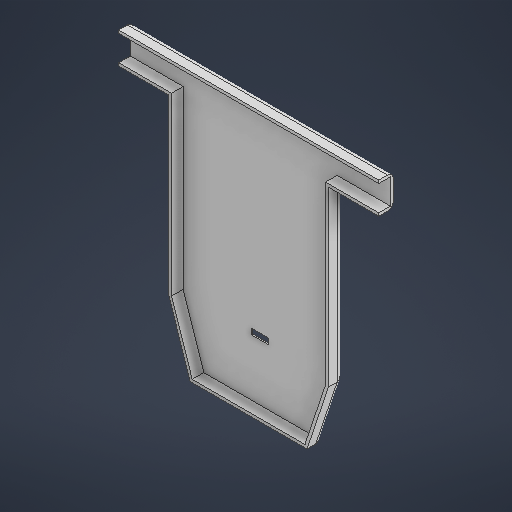
# Autodesk Inventor part: 8.7_수정본
Saved by Autodesk Inventor 2026 (Build 300175000, 175)
## iProperties
Created: 2025-08-07
Part Number: 8.7_수정본
Material: 일반
Document SubType Name: Modeling
Designer: rlarj
Density: 1 g/cm^3
Appearance: 기본값
Author: rlarj
Autodesk Inventor part; units mm, degrees
ref_plane "YZ Plane" through (0, 0, 0) normal (1, 0, 0) x (0, 1, 0)
ref_plane "XZ Plane" through (0, 0, 0) normal (0, 1, 0) x (-1, 0, 0)
ref_plane "XY Plane" through (0, 0, 0) normal (0, 0, 1) x (1, 0, 0)
sketch "스케치18" plane through (0, 0, 0) normal (0, 0, 1) x (1, 0, 0)
  line L0 (55, 0) -> (55, 20)
  line L1 (55, 20) -> (89.63, 20)
  line L2 (89.63, 20) -> (89.63, 41.5)
  line L3 (89.63, 41.5) -> (-89.4, 41.5)
  line L4 (-89.4, 41.5) -> (-89.4, 20)
  line L5 (-89.4, 20) -> (-55, 20)
  line L6 (-55, 20) -> (-55, -55)
  line L7 (55, 0) -> (55, -55)
  line L8 (-55, -55) -> (-55, -99.24)
  line L9 (-55, -99.24) -> (-40.255, -143.4879)
  line L10 (-40.255, -143.4879) -> (40.245, -143.4879)
  line L11 (55, -55) -> (55, -99.24)
  line L12 (55, -99.24) -> (40.245, -143.4879)
  point P0 (0, 0)
  dimension "d111" = 179.03
  dimension "d112" = 184.9879
  dimension "d113" = 34.4
  constraints: 26 end point, 5 vertical, 4 perpendicular, 2 point on line, 1 horizontal
  measures "d111" distance of L2.end L3.end
  measures "d112" vertical distance of L9.end L3.end
  measures "d113" distance of L4.end L5.end
extrude "돌출13" add sketch "스케치18" along normal blind 10
shell "쉘4" thickness 2 removed faces 1 at (-18.3333, -11.6667, 10)
sketch "스케치23" plane through (87.63, 22, 2) normal (-1, 0, 0) x (0, 0, 1)
  line L0 (0, 0) -> (8, 0) projected
  line L1 (0, 0) -> (0, 17.5) projected
  line L2 (8, 0) -> (0, 0)
  line L3 (0, 0) -> (0, 17.5)
  line L4 (0, 17.5) -> (8, 17.5)
  line L5 (8, 17.5) -> (8, 0)
  point P0 (-2, -22)
  constraints: 8 end point, 3 perpendicular, 1 collinear
extrude "돌출16" cut sketch "스케치23" along normal mid plane 600
fillet "모깎기6" radius 4 8 edges at (0.115, 41.5, 0) (72.315, 20, 0) (-72.2, 20, 0) (-55, -39.62, 0) (55, -39.62, 0) (47.6225, -121.3639, 0) (-0.005, -143.4879, 0) (-47.6275, -121.3639, 0)
sketch "스케치24" plane through (0, 0, 0) normal (0, 0, -1) x (-1, 0, 0)
  line L0 (0, -98.5907) -> (-13.5, -98.5907)
  line L1 (0, -98.5907) -> (13.5, -98.5907)
  line L2 (-13.5, -98.5907) -> (-13.5, -128.5907)
  line L3 (-13.5, -128.5907) -> (0, -128.5907)
  line L4 (0, -128.5907) -> (13.5, -128.5907)
  line L5 (13.5, -128.5907) -> (13.5, -98.5907)
  line L6 (0, -98.5907) -> (6, -98.5907)
  line L7 (6, -98.5907) -> (6, -102.5907)
  line L8 (6, -102.5907) -> (-6, -102.5907)
  line L9 (-6, -102.5907) -> (-6, -98.5907)
  point P0 (0, 0)
  dimension "d136" = 6
  dimension "d137" = 4
  dimension "d138" = 12
  constraints: 20 end point, 3 horizontal, 3 perpendicular, 3 point on line, 2 vertical
  measures "d136" distance of L0.start L6.end
  measures "d137" distance of L6.end L7.end
  measures "d138" distance of L7.end L8.end
extrude "돌출17" cut sketch "스케치24" against normal blind 1
sketch "스케치25" plane through (0, 0, 1) normal (0, 0, -1) x (-1, 0, 0)
  line L0 (-13.5, -98.5907) -> (13.5, -98.5907) projected
  line L1 (0, -98.5907) -> (6, -98.5907)
  line L2 (6, -98.5907) -> (6, -102.5907)
  line L3 (6, -102.5907) -> (-6, -102.5907)
  line L4 (-6, -102.5907) -> (-6, -98.5907)
  line L5 (-6, -98.5907) -> (0, -98.5907)
  point P0 (0, 0)
  dimension "d139" = 6
  dimension "d140" = 4
  dimension "d141" = 12
  constraints: 10 end point, 2 perpendicular, 2 point on line, 1 collinear, 1 midpoint, 1 vertical
  measures "d139" distance of L1.start L1.end
  measures "d140" distance of L1.end L2.end
  measures "d141" distance of L2.end L3.end
extrude "돌출18" cut sketch "스케치25" against normal blind 2
sketch "스케치26" plane through (0, 0, 0) normal (0, 0, -1) x (-1, 0, 0)
  point P0 (0, 0)
